Autodesk Fusion 360 part; units mm, degrees
(part 4 of 6)
sketch "minisub_split" plane through (0, 0, 0) normal (0, 1, 0) x (1, 0, 0)
  line L0 (140.6375, -31.1) -> (140.6375, -45.1)
  line L1 (169.2125, -12.05) -> (169.2125, -26.05)
  line L2 (135.5875, -31.1) -> (121.5875, -31.1)
  line L3 (64.4375, -45.1) -> (78.4375, -45.1)
  line L4 (97.4875, -31.1) -> (83.4875, -31.1)
  line L5 (164.1625, -26.05) -> (164.1625, -12.05)
  line L6 (140.6375, -45.1) -> (154.6375, -45.1)
  line L7 (78.4375, -31.1) -> (64.4375, -31.1)
  line L8 (150.1625, -12.05) -> (150.1625, -26.05)
  line L9 (59.3875, -45.1) -> (59.3875, -31.1)
  line L10 (135.5875, -45.1) -> (135.5875, -31.1)
  line L11 (212.075, -12.05) -> (212.075, -26.05)
  line L12 (0.1438, -45.1) -> (14.1438, -45.1)
  line L13 (14.1437, -31.1) -> (0.1437, -31.1)
  line L14 (121.5875, -31.1) -> (121.5875, -45.1)
  line L15 (83.4875, -31.1) -> (83.4875, -45.1)
  line L16 (64.4375, -31.1) -> (64.4375, -45.1)
  line L17 (45.3875, -31.1) -> (45.3875, -45.1)
  line L18 (154.6375, -45.1) -> (154.6375, -31.1)
  line L19 (183.2125, -12.05) -> (169.2125, -12.05)
  line L20 (14.1437, -45.1) -> (14.1437, -31.1)
  line L21 (126.0625, -26.05) -> (126.0625, -12.05)
  line L22 (93.0125, -12.05) -> (93.0125, -26.05)
  line L23 (0.1438, -31.1) -> (0.1438, -45.1)
  line L24 (112.0625, -26.05) -> (126.0625, -26.05)
  line L25 (212.075, -26.05) -> (226.075, -26.05)
  line L26 (126.0625, -12.05) -> (112.0625, -12.05)
  line L27 (173.6875, -31.1) -> (159.6875, -31.1)
  line L28 (159.6875, -45.1) -> (173.6875, -45.1)
  line L29 (73.9625, -12.05) -> (73.9625, -26.05)
  line L30 (40.3375, -45.1) -> (40.3375, -31.1)
  line L31 (169.2125, -26.05) -> (183.2125, -26.05)
  line L32 (26.3375, -45.1) -> (40.3375, -45.1)
  line L33 (131.1125, -26.05) -> (145.1125, -26.05)
  line L34 (107.0125, -12.05) -> (93.0125, -12.05)
  line L35 (45.3875, -45.1) -> (59.3875, -45.1)
  line L36 (188.2625, -12.05) -> (188.2625, -26.05)
  line L37 (116.5375, -45.1) -> (116.5375, -31.1)
  line L38 (115.5307, -49.15) -> (115.5307, -64.15)
  line L39 (171.3063, -50.15) -> (157.3063, -50.15)
  line L40 (78.4375, -45.1) -> (78.4375, -31.1)
  line L41 (202.2625, -12.05) -> (188.2625, -12.05)
  line L42 (226.075, -12.05) -> (212.075, -12.05)
  line L43 (145.1125, -12.05) -> (131.1125, -12.05)
  line L44 (226.075, -26.05) -> (226.075, -12.05)
  line L45 (216.8375, -64.15) -> (230.8375, -64.15)
  line L46 (159.6875, -31.1) -> (159.6875, -45.1)
  line L47 (90.3438, -50.15) -> (76.3438, -50.15)
  line L48 (76.3438, -50.15) -> (76.3438, -64.15)
  line L49 (137.9688, -50.15) -> (123.9688, -50.15)
  line L50 (98.7817, -64.15) -> (98.7817, -49.15)
  line L51 (98.7817, -49.15) -> (91.7817, -49.15)
  line L52 (230.8375, -45.1) -> (230.8375, -31.1)
  line L53 (123.9688, -50.15) -> (123.9688, -64.15)
  line L54 (197.7875, -45.1) -> (211.7875, -45.1)
  line L55 (230.8375, -50.15) -> (216.8375, -50.15)
  line L56 (197.7875, -31.1) -> (197.7875, -45.1)
  line L57 (122.5307, -49.15) -> (115.5307, -49.15)
  line L58 (30.8125, -50.15) -> (16.8125, -50.15)
  line L59 (9.3813, -50.15) -> (-4.6187, -50.15)
  line L60 (52.2438, -64.15) -> (52.2438, -50.15)
  line L61 (211.7875, -45.1) -> (211.7875, -31.1)
  line L62 (216.8375, -31.1) -> (216.8375, -45.1)
  line L63 (137.9688, -64.15) -> (137.9688, -50.15)
  line L64 (216.8375, -45.1) -> (230.8375, -45.1)
  line L65 (90.3438, -64.15) -> (90.3438, -50.15)
  line L66 (178.7375, -45.1) -> (192.7375, -45.1)
  line L67 (157.3063, -64.15) -> (171.3063, -64.15)
  line L68 (139.4067, -49.15) -> (139.4067, -64.15)
  line L69 (122.5307, -64.15) -> (122.5307, -49.15)
  line L70 (52.2438, -50.15) -> (38.2438, -50.15)
  line L71 (91.7817, -64.15) -> (98.7817, -64.15)
  line L72 (157.3063, -50.15) -> (157.3063, -64.15)
  line L73 (211.7875, -31.1) -> (197.7875, -31.1)
  line L74 (139.4067, -64.15) -> (146.4067, -64.15)
  line L75 (74.9058, -64.15) -> (74.9058, -49.15)
  line L76 (-4.6187, -64.15) -> (9.3813, -64.15)
  line L77 (178.7375, -31.1) -> (178.7375, -45.1)
  line L78 (67.9058, -49.15) -> (67.9058, -64.15)
  line L79 (178.7375, -64.15) -> (192.7375, -64.15)
  line L80 (197.7875, -64.15) -> (211.7875, -64.15)
  line L81 (211.7875, -50.15) -> (197.7875, -50.15)
  line L82 (211.7875, -64.15) -> (211.7875, -50.15)
  line L83 (74.9058, -49.15) -> (67.9058, -49.15)
  line L84 (38.2437, -64.15) -> (52.2438, -64.15)
  line L85 (192.7375, -31.1) -> (178.7375, -31.1)
  line L86 (192.7375, -45.1) -> (192.7375, -31.1)
  line L87 (16.8125, -64.15) -> (30.8125, -64.15)
  line L88 (171.3063, -64.15) -> (171.3063, -50.15)
  line L89 (192.7375, -50.15) -> (178.7375, -50.15)
  line L90 (230.8375, -31.1) -> (216.8375, -31.1)
  line L91 (16.8125, -50.15) -> (16.8125, -64.15)
  line L92 (67.9058, -64.15) -> (74.9058, -64.15)
  line L93 (192.7375, -64.15) -> (192.7375, -50.15)
  line L94 (123.9688, -64.15) -> (137.9688, -64.15)
  line L95 (9.3813, -64.15) -> (9.3813, -50.15)
  line L96 (178.7375, -50.15) -> (178.7375, -64.15)
  line L97 (173.6875, -45.1) -> (173.6875, -31.1)
  line L98 (91.7817, -49.15) -> (91.7817, -64.15)
  line L99 (146.4067, -49.15) -> (139.4067, -49.15)
  line L100 (146.4067, -64.15) -> (146.4067, -49.15)
  line L101 (115.5307, -64.15) -> (122.5307, -64.15)
  line L102 (76.3438, -64.15) -> (90.3438, -64.15)
  line L103 (230.8375, -64.15) -> (230.8375, -50.15)
  line L104 (-4.6187, -50.15) -> (-4.6187, -64.15)
  line L105 (216.8375, -50.15) -> (216.8375, -64.15)
  line L106 (197.7875, -50.15) -> (197.7875, -64.15)
  line L107 (38.2437, -50.15) -> (38.2437, -64.15)
  line L108 (30.8125, -64.15) -> (30.8125, -50.15)
  line L109 (-7, 7) -> (-7, -7)
  line L110 (31.1, 7) -> (31.1, -7)
  line L111 (121.3, 7) -> (107.3, 7)
  line L112 (107.3, 7) -> (107.3, -7)
  line L113 (69.2, -7) -> (83.2, -7)
  line L114 (102.25, 7) -> (88.25, 7)
  line L115 (107.3, -7) -> (121.3, -7)
  line L116 (145.4, 7) -> (145.4, -7)
  line L117 (12.05, 7) -> (12.05, -7)
  line L118 (50.15, -7) -> (64.15, -7)
  line L119 (64.15, 7) -> (50.15, 7)
  line L120 (26.05, -7) -> (26.05, 7)
  line L121 (26.05, 7) -> (12.05, 7)
  line L122 (64.15, -7) -> (64.15, 7)
  line L123 (45.1, 7) -> (31.1, 7)
  line L124 (121.3, -7) -> (121.3, 7)
  line L125 (140.35, -7) -> (140.35, 7)
  line L126 (159.4, 7) -> (145.4, 7)
  line L127 (88.25, 7) -> (88.25, -7)
  line L128 (7, -7) -> (7, 7)
  line L129 (50.15, 7) -> (50.15, -7)
  line L130 (178.45, 7) -> (164.45, 7)
  line L131 (126.35, -7) -> (140.35, -7)
  line L132 (12.05, -7) -> (26.05, -7)
  line L133 (-7, -7) -> (7, -7)
  line L134 (45.1, -7) -> (45.1, 7)
  line L135 (140.35, 7) -> (126.35, 7)
  line L136 (69.2, 7) -> (69.2, -7)
  line L137 (164.45, 7) -> (164.45, -7)
  line L138 (159.4, -7) -> (159.4, 7)
  line L139 (83.2, -7) -> (83.2, 7)
  line L140 (178.45, -7) -> (178.45, 7)
  line L141 (145.4, -7) -> (159.4, -7)
  line L142 (183.5, -7) -> (197.5, -7)
  line L143 (126.35, 7) -> (126.35, -7)
  line L144 (164.45, -7) -> (178.45, -7)
  line L145 (7, 7) -> (-7, 7)
  line L146 (88.25, -7) -> (102.25, -7)
  line L147 (31.1, -7) -> (45.1, -7)
  line L148 (102.25, -7) -> (102.25, 7)
  line L149 (83.2, 7) -> (69.2, 7)
  line L150 (183.5, 7) -> (183.5, -7)
  line L151 (209.6937, -7) -> (223.6938, -7)
  line L152 (223.6938, 7) -> (209.6937, 7)
  line L153 (223.6938, -7) -> (223.6938, 7)
  line L154 (209.6937, 7) -> (209.6937, -7)
  line L155 (197.5, 7) -> (183.5, 7)
  line L156 (197.5, -7) -> (197.5, 7)
  line L157 (-4.6187, -12.05) -> (-4.6187, -26.05)
  line L158 (16.8125, -26.05) -> (30.8125, -26.05)
  line L159 (30.8125, -12.05) -> (16.8125, -12.05)
  line L160 (30.8125, -26.05) -> (30.8125, -12.05)
  line L161 (35.8625, -26.05) -> (49.8625, -26.05)
  line L162 (35.8625, -12.05) -> (35.8625, -26.05)
  line L163 (68.9125, -26.05) -> (68.9125, -12.05)
  line L164 (54.9125, -12.05) -> (54.9125, -26.05)
  line L165 (73.9625, -26.05) -> (87.9625, -26.05)
  line L166 (49.8625, -26.05) -> (49.8625, -12.05)
  line L167 (68.9125, -12.05) -> (54.9125, -12.05)
  line L168 (54.9125, -26.05) -> (68.9125, -26.05)
  line L169 (9.3813, -12.05) -> (-4.6187, -12.05)
  line L170 (16.8125, -12.05) -> (16.8125, -26.05)
  line L171 (49.8625, -12.05) -> (35.8625, -12.05)
  line L172 (87.9625, -12.05) -> (73.9625, -12.05)
  line L173 (-4.6187, -26.05) -> (9.3813, -26.05)
  line L174 (9.3813, -26.05) -> (9.3813, -12.05)
  line L175 (107.0125, -26.05) -> (107.0125, -12.05)
  line L176 (202.2625, -26.05) -> (202.2625, -12.05)
  line L177 (26.3375, -31.1) -> (26.3375, -45.1)
  line L178 (150.1625, -26.05) -> (164.1625, -26.05)
  line L179 (83.4875, -45.1) -> (97.4875, -45.1)
  line L180 (121.5875, -45.1) -> (135.5875, -45.1)
  line L181 (183.2125, -26.05) -> (183.2125, -12.05)
  line L182 (154.6375, -31.1) -> (140.6375, -31.1)
  line L183 (131.1125, -12.05) -> (131.1125, -26.05)
  line L184 (112.0625, -12.05) -> (112.0625, -26.05)
  line L185 (40.3375, -31.1) -> (26.3375, -31.1)
  line L186 (102.5375, -45.1) -> (116.5375, -45.1)
  line L187 (97.4875, -45.1) -> (97.4875, -31.1)
  line L188 (87.9625, -26.05) -> (87.9625, -12.05)
  line L189 (93.0125, -26.05) -> (107.0125, -26.05)
  line L190 (102.5375, -31.1) -> (102.5375, -45.1)
  line L191 (116.5375, -31.1) -> (102.5375, -31.1)
  line L192 (145.1125, -26.05) -> (145.1125, -12.05)
  line L193 (188.2625, -26.05) -> (202.2625, -26.05)
  line L194 (59.3875, -31.1) -> (45.3875, -31.1)
  line L195 (164.1625, -12.05) -> (150.1625, -12.05)
sketch "m3n3van_r2" plane through (0, 0, 0) normal (0, 1, 0) x (1, 0, 0)
  line L0 (159.4, 7) -> (145.4, 7)
  line L1 (159.4, -7) -> (159.4, 7)
  line L2 (7, -7) -> (7, 7)
  line L3 (164.45, -7) -> (178.45, -7)
  line L4 (178.45, -7) -> (178.45, 7)
  line L5 (26.05, 7) -> (12.05, 7)
  line L6 (183.5, -7) -> (197.5, -7)
  line L7 (164.45, 7) -> (164.45, -7)
  line L8 (50.15, 7) -> (50.15, -7)
  line L9 (88.25, -7) -> (102.25, -7)
  line L10 (83.2, -7) -> (83.2, 7)
  line L11 (69.2, -7) -> (83.2, -7)
  line L12 (107.3, -7) -> (121.3, -7)
  line L13 (121.3, 7) -> (107.3, 7)
  line L14 (121.3, -7) -> (121.3, 7)
  line L15 (145.4, -7) -> (159.4, -7)
  line L16 (31.1, -7) -> (45.1, -7)
  line L17 (-7, 7) -> (-7, -7)
  line L18 (45.1, 7) -> (31.1, 7)
  line L19 (45.1, -7) -> (45.1, 7)
  line L20 (7, 7) -> (-7, 7)
  line L21 (12.05, 7) -> (12.05, -7)
  line L22 (178.45, 7) -> (164.45, 7)
  line L23 (145.4, 7) -> (145.4, -7)
  line L24 (26.05, -7) -> (26.05, 7)
  line L25 (102.25, 7) -> (88.25, 7)
  line L26 (50.15, -7) -> (64.15, -7)
  line L27 (126.35, 7) -> (126.35, -7)
  line L28 (-7, -7) -> (7, -7)
  line L29 (31.1, 7) -> (31.1, -7)
  line L30 (12.05, -7) -> (26.05, -7)
  line L31 (140.35, 7) -> (126.35, 7)
  line L32 (93.0125, -12.05) -> (93.0125, -26.05)
  line L33 (169.2125, -26.05) -> (183.2125, -26.05)
  line L34 (9.3812, -26.05) -> (9.3812, -12.05)
  line L35 (219.2187, -7) -> (223.6937, -7)
  line L36 (30.8125, -12.05) -> (16.8125, -12.05)
  line L37 (126.0625, -26.05) -> (126.0625, -12.05)
  line L38 (112.0625, -26.05) -> (126.0625, -26.05)
  line L39 (145.1125, -26.05) -> (145.1125, -12.05)
  line L40 (126.0625, -12.05) -> (112.0625, -12.05)
  line L41 (140.35, -7) -> (140.35, 7)
  line L42 (102.25, -7) -> (102.25, 7)
  line L43 (183.5, 7) -> (183.5, -7)
  line L44 (145.1125, -12.05) -> (131.1125, -12.05)
  line L45 (212.075, -26.05) -> (226.075, -26.05)
  line L46 (232.5253, 7) -> (223.6937, 7)
  line L47 (68.9125, -26.05) -> (68.9125, -12.05)
  line L48 (107.0125, -26.05) -> (107.0125, -12.05)
  line L49 (197.5, -7) -> (197.5, 7)
  line L50 (209.6937, -7) -> (216.55, -7)
  line L51 (49.8625, -12.05) -> (35.8625, -12.05)
  line L52 (83.2, 7) -> (69.2, 7)
  line L53 (107.0125, -12.05) -> (93.0125, -12.05)
  line L54 (164.1625, -12.05) -> (150.1625, -12.05)
  line L55 (150.1625, -12.05) -> (150.1625, -26.05)
  line L56 (223.6937, -7) -> (232.5253, -7)
  line L57 (188.2625, -26.05) -> (202.2625, -26.05)
  line L58 (16.8125, -12.05) -> (16.8125, -26.05)
  line L59 (223.6937, 7) -> (219.2187, 7)
  line L60 (209.6937, 7) -> (202.55, 7)
  line L61 (68.9125, -12.05) -> (54.9125, -12.05)
  line L62 (126.35, -7) -> (140.35, -7)
  line L63 (219.2187, 7) -> (216.55, 7)
  line L64 (216.55, 7) -> (209.6937, 7)
  line L65 (35.8625, -26.05) -> (49.8625, -26.05)
  line L66 (30.8125, -26.05) -> (30.8125, -12.05)
  line L67 (73.9625, -26.05) -> (87.9625, -26.05)
  line L68 (-4.6187, -12.05) -> (-4.6187, -26.05)
  line L69 (54.9125, -26.05) -> (68.9125, -26.05)
  line L70 (202.55, 7) -> (202.55, -7)
  line L71 (169.2125, -12.05) -> (169.2125, -26.05)
  line L72 (202.2625, -26.05) -> (202.2625, -12.05)
  line L73 (49.8625, -26.05) -> (49.8625, -12.05)
  line L74 (112.0625, -12.05) -> (112.0625, -26.05)
  line L75 (131.1125, -26.05) -> (145.1125, -26.05)
  line L76 (131.1125, -12.05) -> (131.1125, -26.05)
  line L77 (107.3, 7) -> (107.3, -7)
  line L78 (216.55, -7) -> (219.2187, -7)
  line L79 (-4.6187, -26.05) -> (9.3812, -26.05)
  line L80 (16.8125, -26.05) -> (30.8125, -26.05)
  line L81 (54.9125, -12.05) -> (54.9125, -26.05)
  line L82 (64.15, -7) -> (64.15, 7)
  line L83 (197.5, 7) -> (183.5, 7)
  line L84 (64.15, 7) -> (50.15, 7)
  line L85 (87.9625, -26.05) -> (87.9625, -12.05)
  line L86 (35.8625, -12.05) -> (35.8625, -26.05)
  line L87 (202.2625, -12.05) -> (188.2625, -12.05)
  line L88 (183.2125, -12.05) -> (169.2125, -12.05)
  line L89 (183.2125, -26.05) -> (183.2125, -12.05)
  line L90 (9.3812, -12.05) -> (-4.6187, -12.05)
  line L91 (188.2625, -12.05) -> (188.2625, -26.05)
  line L92 (88.25, 7) -> (88.25, -7)
  line L93 (202.55, -7) -> (209.6937, -7)
  line L94 (69.2, 7) -> (69.2, -7)
  line L95 (232.5253, -7) -> (232.5253, 7)
  line L96 (87.9625, -12.05) -> (73.9625, -12.05)
  line L97 (64.4375, -31.1) -> (64.4375, -45.1)
  line L98 (216.8375, -31.1) -> (216.8375, -45.1)
  line L99 (14.1437, -45.1) -> (14.1437, -31.1)
  line L100 (14.4313, -64.15) -> (28.4312, -64.15)
  line L101 (40.3375, -31.1) -> (26.3375, -31.1)
  line L102 (59.3875, -31.1) -> (45.3875, -31.1)
  line L103 (102.5375, -45.1) -> (116.5375, -45.1)
  line L104 (230.8375, -45.1) -> (230.8375, -31.1)
  line L105 (164.1625, -26.05) -> (164.1625, -12.05)
  line L106 (121.5875, -31.1) -> (121.5875, -45.1)
  line L107 (7, -50.15) -> (-7, -50.15)
  line L108 (116.5375, -31.1) -> (102.5375, -31.1)
  line L109 (211.7875, -45.1) -> (211.7875, -31.1)
  line L110 (28.4312, -50.15) -> (14.4313, -50.15)
  line L111 (140.6375, -45.1) -> (154.6375, -45.1)
  line L112 (102.5375, -31.1) -> (102.5375, -45.1)
  line L113 (135.5875, -31.1) -> (121.5875, -31.1)
  line L114 (14.4313, -50.15) -> (14.4313, -64.15)
  line L115 (26.3375, -31.1) -> (26.3375, -45.1)
  line L116 (78.4375, -31.1) -> (64.4375, -31.1)
  line L117 (192.7375, -31.1) -> (178.7375, -31.1)
  line L118 (73.9625, -12.05) -> (73.9625, -26.05)
  line L119 (197.7875, -45.1) -> (211.7875, -45.1)
  line L120 (78.4375, -45.1) -> (78.4375, -31.1)
  line L121 (28.4312, -64.15) -> (28.4312, -50.15)
  line L122 (0.1438, -31.1) -> (0.1438, -45.1)
  line L123 (73.9625, -64.15) -> (87.9625, -64.15)
  line L124 (159.6875, -31.1) -> (159.6875, -45.1)
  line L125 (150.1625, -26.05) -> (164.1625, -26.05)
  line L126 (173.6875, -45.1) -> (173.6875, -31.1)
  line L127 (226.075, -26.05) -> (226.075, -12.05)
  line L128 (197.7875, -31.1) -> (197.7875, -45.1)
  line L129 (14.1437, -31.1) -> (0.1438, -31.1)
  line L130 (35.8625, -50.15) -> (35.8625, -64.15)
  line L131 (49.8625, -64.15) -> (49.8625, -50.15)
  line L132 (97.4875, -31.1) -> (83.4875, -31.1)
  line L133 (97.4875, -45.1) -> (97.4875, -31.1)
  line L134 (121.5875, -45.1) -> (135.5875, -45.1)
  line L135 (35.8625, -64.15) -> (49.8625, -64.15)
  line L136 (226.075, -12.05) -> (212.075, -12.05)
  line L137 (173.6875, -31.1) -> (159.6875, -31.1)
  line L138 (211.7875, -31.1) -> (197.7875, -31.1)
  line L139 (192.7375, -45.1) -> (192.7375, -31.1)
  line L140 (49.8625, -50.15) -> (35.8625, -50.15)
  line L141 (64.4375, -45.1) -> (78.4375, -45.1)
  line L142 (-7, -50.15) -> (-7, -64.15)
  line L143 (93.0125, -26.05) -> (107.0125, -26.05)
  line L144 (83.4875, -31.1) -> (83.4875, -45.1)
  line L145 (154.6375, -45.1) -> (154.6375, -31.1)
  line L146 (26.3375, -45.1) -> (40.3375, -45.1)
  line L147 (45.3875, -45.1) -> (59.3875, -45.1)
  line L148 (45.3875, -31.1) -> (45.3875, -45.1)
  line L149 (116.5375, -45.1) -> (116.5375, -31.1)
  line L150 (83.4875, -45.1) -> (97.4875, -45.1)
  line L151 (154.6375, -31.1) -> (140.6375, -31.1)
  line L152 (230.8375, -31.1) -> (216.8375, -31.1)
  line L153 (178.7375, -45.1) -> (192.7375, -45.1)
  line L154 (7, -64.15) -> (7, -50.15)
  line L155 (178.7375, -31.1) -> (178.7375, -45.1)
  line L156 (0.1438, -45.1) -> (14.1437, -45.1)
  line L157 (216.8375, -45.1) -> (230.8375, -45.1)
  line L158 (212.075, -12.05) -> (212.075, -26.05)
  line L159 (140.6375, -31.1) -> (140.6375, -45.1)
  line L160 (-7, -64.15) -> (7, -64.15)
  line L161 (115.5625, -64.15) -> (122.5625, -64.15)
  line L162 (87.9625, -64.15) -> (87.9625, -50.15)
  line L163 (185.5937, -50.15) -> (171.5937, -50.15)
  line L164 (214.4562, -50.15) -> (214.4562, -64.15)
  line L165 (131.1125, -50.15) -> (131.1125, -64.15)
  line L166 (171.5937, -50.15) -> (171.5937, -64.15)
  line L167 (207.025, -50.15) -> (193.025, -50.15)
  line L168 (65.4125, -49.15) -> (58.4125, -49.15)
  line L169 (115.5625, -49.15) -> (115.5625, -64.15)
  line L170 (228.4562, -64.15) -> (228.4562, -50.15)
  line L171 (160.6625, -64.15) -> (160.6625, -49.15)
  line L172 (103.5125, -64.15) -> (103.5125, -49.15)
  line L173 (145.1125, -64.15) -> (145.1125, -50.15)
  line L174 (193.025, -64.15) -> (207.025, -64.15)
  line L175 (59.3875, -45.1) -> (59.3875, -31.1)
  line L176 (122.5625, -49.15) -> (115.5625, -49.15)
  line L177 (145.1125, -50.15) -> (131.1125, -50.15)
  line L178 (103.5125, -49.15) -> (96.5125, -49.15)
  line L179 (131.1125, -64.15) -> (145.1125, -64.15)
  line L180 (159.6875, -45.1) -> (173.6875, -45.1)
  line L181 (40.3375, -45.1) -> (40.3375, -31.1)
  line L182 (135.5875, -45.1) -> (135.5875, -31.1)
  line L183 (160.6625, -49.15) -> (153.6625, -49.15)
  line L184 (96.5125, -64.15) -> (103.5125, -64.15)
  line L185 (171.5937, -64.15) -> (185.5937, -64.15)
  line L186 (193.025, -50.15) -> (193.025, -64.15)
  line L187 (214.4562, -64.15) -> (228.4562, -64.15)
  line L188 (65.4125, -64.15) -> (65.4125, -49.15)
  line L189 (122.5625, -64.15) -> (122.5625, -49.15)
  line L190 (185.5937, -64.15) -> (185.5937, -50.15)
  line L191 (73.9625, -50.15) -> (73.9625, -64.15)
  line L192 (96.5125, -49.15) -> (96.5125, -64.15)
  line L193 (87.9625, -50.15) -> (73.9625, -50.15)
  line L194 (153.6625, -49.15) -> (153.6625, -64.15)
  line L195 (228.4562, -50.15) -> (214.4562, -50.15)
  line L196 (153.6625, -64.15) -> (160.6625, -64.15)
  line L197 (58.4125, -64.15) -> (65.4125, -64.15)
  line L198 (207.025, -64.15) -> (207.025, -50.15)
  line L199 (58.4125, -49.15) -> (58.4125, -64.15)
sketch "asymptote" plane through (0, 0, 0) normal (0, 1, 0) x (1, 0, 0)
  line L0 (54.9125, -26.05) -> (54.9125, -12.05)
  line L1 (97.4875, -31.1) -> (97.4875, -45.1)
  line L2 (97.4875, -45.1) -> (83.4875, -45.1)
  line L3 (83.4875, -45.1) -> (83.4875, -31.1)
  line L4 (71.2938, -64.15) -> (57.2938, -64.15)
  line L5 (107.3, 7) -> (121.3, 7)
  line L6 (121.3, 7) -> (121.3, -7)
  line L7 (121.3, -7) -> (107.3, -7)
  line L8 (107.3, -7) -> (107.3, 7)
  line L9 (145.1125, -12.05) -> (145.1125, -26.05)
  line L10 (57.2938, -64.15) -> (57.2938, -50.15)
  line L11 (145.1125, -26.05) -> (131.1125, -26.05)
  line L12 (131.1125, -26.05) -> (131.1125, -12.05)
  line L13 (58.4125, -49.15) -> (65.4125, -49.15)
  line L14 (7, 7) -> (7, -7)
  line L15 (40.3375, -31.1) -> (40.3375, -45.1)
  line L16 (26.3375, -31.1) -> (40.3375, -31.1)
  line L17 (54.9125, -12.05) -> (68.9125, -12.05)
  line L18 (68.9125, -12.05) -> (68.9125, -26.05)
  line L19 (40.3375, -45.1) -> (26.3375, -45.1)
  line L20 (71.2938, -50.15) -> (71.2938, -64.15)
  line L21 (57.2938, -50.15) -> (58.4125, -50.15)
  line L22 (65.4125, -50.15) -> (71.2938, -50.15)
  line L23 (65.4125, -49.15) -> (65.4125, -50.15)
  line L24 (26.3375, -45.1) -> (26.3375, -31.1)
  line L25 (7, -7) -> (-7, -7)
  line L26 (-7, -7) -> (-7, 7)
  line L27 (68.9125, -26.05) -> (54.9125, -26.05)
  line L28 (58.4125, -50.15) -> (58.4125, -49.15)
  line L29 (-7, 7) -> (7, 7)
  line L30 (83.4875, -31.1) -> (97.4875, -31.1)
  line L31 (50.15, 7) -> (64.15, 7)
  line L32 (230.8375, -31.1) -> (230.8375, -45.1)
  line L33 (-4.6187, -12.05) -> (9.3812, -12.05)
  line L34 (49.8625, -12.05) -> (49.8625, -26.05)
  line L35 (226.075, -12.05) -> (226.075, -26.05)
  line L36 (188.2625, -12.05) -> (202.2625, -12.05)
  line L37 (9.3812, -26.05) -> (-4.6187, -26.05)
  line L38 (50.15, -7) -> (50.15, 7)
  line L39 (192.7375, -45.1) -> (178.7375, -45.1)
  line L40 (88.25, -7) -> (88.25, 7)
  line L41 (159.6875, -45.1) -> (159.6875, -31.1)
  line L42 (9.3812, -12.05) -> (9.3812, -26.05)
  line L43 (-4.6187, -26.05) -> (-4.6187, -12.05)
  line L44 (37.9563, -64.15) -> (-2.2375, -64.15)
  line L45 (226.075, -26.05) -> (212.075, -26.05)
  line L46 (230.8375, -45.1) -> (216.8375, -45.1)
  line L47 (183.2125, -12.05) -> (183.2125, -26.05)
  line L48 (103.5125, -49.15) -> (103.5125, -50.15)
  line L49 (88.25, 7) -> (102.25, 7)
  line L50 (216.8375, -31.1) -> (230.8375, -31.1)
  line L51 (192.7375, -31.1) -> (192.7375, -45.1)
  line L52 (173.6875, -45.1) -> (159.6875, -45.1)
  line L53 (131.1125, -12.05) -> (145.1125, -12.05)
  line L54 (159.6875, -31.1) -> (173.6875, -31.1)
  line L55 (173.6875, -31.1) -> (173.6875, -45.1)
  line L56 (178.7375, -31.1) -> (192.7375, -31.1)
  line L57 (212.075, -26.05) -> (212.075, -12.05)
  line L58 (188.2625, -26.05) -> (188.2625, -12.05)
  line L59 (64.15, 7) -> (64.15, -7)
  line L60 (32.1068, -50.15) -> (37.9563, -50.15)
  line L61 (73.9625, -64.15) -> (73.9625, -50.15)
  line L62 (169.2125, -26.05) -> (169.2125, -12.05)
  line L63 (12.05, 7) -> (26.05, 7)
  line L64 (26.05, 7) -> (26.05, -7)
  line L65 (25.1068, -50.15) -> (25.1068, -49.15)
  line L66 (64.4375, -31.1) -> (78.4375, -31.1)
  line L67 (32.1068, -49.15) -> (32.1068, -50.15)
  line L68 (-2.2375, -64.15) -> (-2.2375, -50.15)
  line L69 (122.5625, -49.15) -> (122.5625, -50.15)
  line L70 (145.1125, -50.15) -> (145.1125, -64.15)
  line L71 (216.8375, -45.1) -> (216.8375, -31.1)
  line L72 (178.7375, -45.1) -> (178.7375, -31.1)
  line L73 (212.075, -12.05) -> (226.075, -12.05)
  line L74 (-2.2375, -50.15) -> (1.2308, -50.15)
  line L75 (202.2625, -12.05) -> (202.2625, -26.05)
  line L76 (202.2625, -26.05) -> (188.2625, -26.05)
  line L77 (140.6375, -45.1) -> (140.6375, -31.1)
  line L78 (64.15, -7) -> (50.15, -7)
  line L79 (8.2307, -50.15) -> (25.1068, -50.15)
  line L80 (112.0625, -26.05) -> (112.0625, -12.05)
  line L81 (35.8625, -12.05) -> (49.8625, -12.05)
  line L82 (1.2308, -49.15) -> (8.2307, -49.15)
  line L83 (122.5625, -50.15) -> (145.1125, -50.15)
  line L84 (169.2125, -12.05) -> (183.2125, -12.05)
  line L85 (73.9625, -50.15) -> (96.5125, -50.15)
  line L86 (35.8625, -26.05) -> (35.8625, -12.05)
  line L87 (83.2, 7) -> (83.2, -7)
  line L88 (96.5125, -50.15) -> (96.5125, -49.15)
  line L89 (1.2308, -50.15) -> (1.2308, -49.15)
  line L90 (78.4375, -45.1) -> (64.4375, -45.1)
  line L91 (96.5125, -49.15) -> (103.5125, -49.15)
  line L92 (140.6375, -31.1) -> (154.6375, -31.1)
  line L93 (126.0625, -26.05) -> (112.0625, -26.05)
  line L94 (83.2, -7) -> (69.2, -7)
  line L95 (145.4, -7) -> (145.4, 7)
  line L96 (197.5, 7) -> (197.5, -7)
  line L97 (197.7875, -45.1) -> (197.7875, -31.1)
  line L98 (37.9563, -50.15) -> (37.9563, -64.15)
  line L99 (145.1125, -64.15) -> (73.9625, -64.15)
  line L100 (78.4375, -31.1) -> (78.4375, -45.1)
  line L101 (14.1437, -31.1) -> (14.1437, -45.1)
  line L102 (49.8625, -26.05) -> (35.8625, -26.05)
  line L103 (112.0625, -12.05) -> (126.0625, -12.05)
  line L104 (107.0125, -26.05) -> (93.0125, -26.05)
  line L105 (189.2375, -49.15) -> (189.2375, -50.15)
  line L106 (8.2307, -49.15) -> (8.2307, -50.15)
  line L107 (183.2125, -26.05) -> (169.2125, -26.05)
  line L108 (64.4375, -45.1) -> (64.4375, -31.1)
  line L109 (0.1438, -45.1) -> (0.1438, -31.1)
  line L110 (93.0125, -26.05) -> (93.0125, -12.05)
  line L111 (154.6375, -45.1) -> (140.6375, -45.1)
  line L112 (154.6375, -31.1) -> (154.6375, -45.1)
  line L113 (126.0625, -12.05) -> (126.0625, -26.05)
  line L114 (12.05, -7) -> (12.05, 7)
  line L115 (227.3375, -50.15) -> (230.8375, -50.15)
  line L116 (126.35, -7) -> (126.35, 7)
  line L117 (26.05, -7) -> (12.05, -7)
  line L118 (209.6938, -7) -> (209.6938, 7)
  line L119 (140.35, -7) -> (126.35, -7)
  line L120 (69.2, 7) -> (83.2, 7)
  line L121 (0.1438, -31.1) -> (14.1437, -31.1)
  line L122 (14.1437, -45.1) -> (0.1438, -45.1)
  line L123 (115.5625, -50.15) -> (115.5625, -49.15)
  line L124 (103.5125, -50.15) -> (115.5625, -50.15)
  line L125 (25.1068, -49.15) -> (32.1068, -49.15)
  line L126 (102.25, -7) -> (88.25, -7)
  line L127 (115.5625, -49.15) -> (122.5625, -49.15)
  line L128 (102.5375, -45.1) -> (102.5375, -31.1)
  line L129 (102.25, 7) -> (102.25, -7)
  line L130 (164.1625, -26.05) -> (150.1625, -26.05)
  line L131 (211.7875, -31.1) -> (211.7875, -45.1)
  line L132 (116.5375, -45.1) -> (102.5375, -45.1)
  line L133 (211.7875, -45.1) -> (197.7875, -45.1)
  line L134 (223.6938, 7) -> (223.6938, -7)
  line L135 (178.7375, -50.15) -> (182.2375, -50.15)
  line L136 (159.4, 7) -> (159.4, -7)
  line L137 (150.1625, -26.05) -> (150.1625, -12.05)
  line L138 (182.2375, -50.15) -> (182.2375, -49.15)
  line L139 (31.1, -7) -> (31.1, 7)
  line L140 (189.2375, -50.15) -> (220.3375, -50.15)
  line L141 (220.3375, -50.15) -> (220.3375, -49.15)
  line L142 (230.8375, -50.15) -> (230.8375, -64.15)
  line L143 (178.45, 7) -> (178.45, -7)
  line L144 (135.5875, -31.1) -> (135.5875, -45.1)
  line L145 (87.9625, -26.05) -> (73.9625, -26.05)
  line L146 (182.2375, -49.15) -> (189.2375, -49.15)
  line L147 (45.1, 7) -> (45.1, -7)
  line L148 (102.5375, -31.1) -> (116.5375, -31.1)
  line L149 (178.7375, -64.15) -> (178.7375, -50.15)
  line L150 (150.1625, -12.05) -> (164.1625, -12.05)
  line L151 (69.2, -7) -> (69.2, 7)
  line L152 (73.9625, -12.05) -> (87.9625, -12.05)
  line L153 (178.45, -7) -> (164.45, -7)
  line L154 (197.7875, -31.1) -> (211.7875, -31.1)
  line L155 (230.8375, -64.15) -> (178.7375, -64.15)
  line L156 (164.45, -7) -> (164.45, 7)
  line L157 (209.6938, 7) -> (223.6938, 7)
  line L158 (183.5, -7) -> (183.5, 7)
  line L159 (220.3375, -49.15) -> (227.3375, -49.15)
  line L160 (45.1, -7) -> (31.1, -7)
  line L161 (31.1, 7) -> (45.1, 7)
  line L162 (87.9625, -12.05) -> (87.9625, -26.05)
  line L163 (183.5, 7) -> (197.5, 7)
  line L164 (223.6938, -7) -> (209.6938, -7)
  line L165 (121.5875, -31.1) -> (135.5875, -31.1)
  line L166 (93.0125, -12.05) -> (107.0125, -12.05)
  line L167 (227.3375, -49.15) -> (227.3375, -50.15)
  line L168 (145.4, 7) -> (159.4, 7)
  line L169 (140.35, 7) -> (140.35, -7)
  line L170 (135.5875, -45.1) -> (121.5875, -45.1)
  line L171 (107.0125, -12.05) -> (107.0125, -26.05)
  line L172 (197.5, -7) -> (183.5, -7)
  line L173 (73.9625, -26.05) -> (73.9625, -12.05)
  line L174 (126.35, 7) -> (140.35, 7)
  line L175 (164.45, 7) -> (178.45, 7)
  line L176 (116.5375, -31.1) -> (116.5375, -45.1)
  line L177 (159.4, -7) -> (145.4, -7)
  line L178 (164.1625, -12.05) -> (164.1625, -26.05)
  line L179 (121.5875, -45.1) -> (121.5875, -31.1)
  line L180 (30.8125, -12.05) -> (30.8125, -26.05)
  line L181 (153.6625, -49.15) -> (160.6625, -49.15)
  line L182 (16.8125, -12.05) -> (30.8125, -12.05)
  line L183 (45.3875, -45.1) -> (45.3875, -31.1)
  line L184 (147.7813, -50.15) -> (153.6625, -50.15)
  line L185 (45.3875, -31.1) -> (59.3875, -31.1)
  line L186 (160.6625, -50.15) -> (161.7813, -50.15)
  line L187 (30.8125, -26.05) -> (16.8125, -26.05)
  line L188 (153.6625, -50.15) -> (153.6625, -49.15)
  line L189 (59.3875, -31.1) -> (59.3875, -45.1)
  line L190 (161.7813, -50.15) -> (161.7813, -64.15)
  line L191 (160.6625, -49.15) -> (160.6625, -50.15)
  line L192 (16.8125, -26.05) -> (16.8125, -12.05)
  line L193 (59.3875, -45.1) -> (45.3875, -45.1)
  line L194 (161.7813, -64.15) -> (147.7813, -64.15)
  line L195 (147.7813, -64.15) -> (147.7813, -50.15)
sketch "asymptote_7u" plane through (35.5023, 0, -36.9816) normal (0, 1, 0) x (1, 0, 0)
  line L0 (81.0349, -96.4308) -> (127.8099, -96.4308)
  line L1 (134.5609, -96.4308) -> (135.3849, -96.4308)
  line L2 (13.5097, -87.3619) -> (13.5097, -93.632)
  line L3 (67.0356, -96.4322) -> (67.0356, -101.1313)
  line L4 (15.235, -86.1616) -> (15.235, -87.3619)
  line L5 (18.5341, -87.3619) -> (18.5341, -86.1616)
  line L6 (135.3849, -96.4308) -> (135.3849, -93.6306)
  line L7 (129.5349, -86.1603) -> (129.5349, -87.3605)
  line L8 (129.5349, -87.3605) -> (127.8099, -87.3605)
  line L9 (132.8349, -87.3605) -> (132.8349, -86.1603)
  line L10 (134.5609, -93.6306) -> (134.5609, -87.3605)
  line L11 (18.5341, -86.1616) -> (15.235, -86.1616)
  line L12 (12.6843, -96.4322) -> (13.5097, -96.4322)
  line L13 (127.8099, -99.6623) -> (134.5609, -99.6623)
  line L14 (134.5609, -87.3605) -> (132.8349, -87.3605)
  line L15 (135.3849, -93.6306) -> (134.5609, -93.6306)
  line L16 (20.2608, -99.6623) -> (20.2608, -96.4322)
  line L17 (127.8099, -87.3605) -> (127.8099, -91.8309)
  line L18 (134.5609, -99.6623) -> (134.5609, -96.4308)
  line L19 (81.0349, -87.1318) -> (67.0356, -87.1318)
  line L20 (12.6843, -93.632) -> (12.6843, -96.4322)
  line L21 (67.0356, -87.1318) -> (67.0356, -91.8323)
  line L22 (13.5097, -93.632) -> (12.6843, -93.632)
  line L23 (20.2608, -87.3619) -> (18.5341, -87.3619)
  line L24 (127.8099, -91.8309) -> (81.0349, -91.8309)
  line L25 (15.235, -87.3619) -> (13.5097, -87.3619)
  line L26 (67.0356, -101.1313) -> (81.0349, -101.1313)
  line L27 (20.2608, -91.8323) -> (20.2608, -87.3619)
  line L28 (132.8349, -86.1603) -> (129.5349, -86.1603)
  line L29 (67.0356, -91.8323) -> (20.2608, -91.8323)
  line L30 (13.5097, -96.4322) -> (13.5097, -99.6623)
  line L31 (81.0349, -101.1313) -> (81.0349, -96.4308)
  line L32 (81.0349, -91.8309) -> (81.0349, -87.1318)
  line L33 (20.2608, -96.4322) -> (67.0356, -96.4322)
  line L34 (127.8099, -96.4308) -> (127.8099, -99.6623)
  line L35 (13.5097, -99.6623) -> (20.2608, -99.6623)
  line L36 (67.0356, -87.1318) -> (81.0349, -101.1313) construction
  line L37 (67.0356, -101.1313) -> (81.0349, -87.1318) construction
sketch "minibaen" plane through (0, 0, 0) normal (0, 1, 0) x (1, 0, 0)
  line L0 (104.919, -31.098) -> (104.919, -45.098)
  line L1 (118.919, -45.098) -> (118.919, -31.098)
  line L2 (67.559, -64.148) -> (68.461, -64.148)
  line L3 (160.959, -31.098) -> (160.959, -45.098)
  line L4 (216.999, -31.098) -> (216.999, -45.098)
  line L5 (86.239, -31.098) -> (86.239, -45.098)
  line L6 (160.959, -45.098) -> (174.959, -45.098)
  line L7 (81.559, -50.148) -> (76.899, -50.148)
  line L8 (90.109, -64.148) -> (90.899, -64.148)
  line L9 (25.519, -64.148) -> (25.519, -50.148)
  line L10 (198.319, -31.098) -> (198.319, -45.098)
  line L11 (230.999, -45.098) -> (230.999, -31.098)
  line L12 (137.599, -50.148) -> (133.729, -50.148)
  line L13 (124.501, -64.148) -> (126.729, -64.148)
  line L14 (172.569, -49.148) -> (171.829, -49.148)
  line L15 (48.879, -64.148) -> (51.269, -64.148)
  line L16 (179.639, -31.098) -> (179.639, -45.098)
  line L17 (148.377, -49.148) -> (148.377, -50.148)
  line L18 (59.009, -64.148) -> (62.879, -64.148)
  line L19 (76.899, -64.148) -> (81.559, -64.148)
  line L20 (52.009, -64.148) -> (58.269, -64.148)
  line L21 (68.461, -50.148) -> (67.559, -50.148)
  line L22 (165.569, -49.148) -> (164.829, -49.148)
  line L23 (118.919, -64.148) -> (118.919, -50.148)
  line L24 (164.829, -64.148) -> (165.569, -64.148)
  line L25 (90.109, -50.148) -> (86.239, -50.148)
  line L26 (86.239, -64.148) -> (90.109, -64.148)
  line L27 (146.939, -64.148) -> (148.377, -64.148)
  line L28 (104.919, -50.148) -> (104.919, -64.148)
  line L29 (97.109, -64.148) -> (99.337, -64.148)
  line L30 (126.729, -49.148) -> (124.501, -49.148)
  line L31 (123.599, -45.098) -> (137.599, -45.098)
  line L32 (193.639, -45.098) -> (193.639, -31.098)
  line L33 (-7.161, -64.148) -> (6.839, -64.148)
  line L34 (58.269, -64.148) -> (59.009, -64.148)
  line L35 (30.199, -50.148) -> (30.199, -64.148)
  line L36 (59.009, -50.148) -> (59.009, -49.148)
  line L37 (212.319, -45.098) -> (212.319, -31.098)
  line L38 (137.599, -45.098) -> (137.599, -31.098)
  line L39 (133.729, -64.148) -> (137.599, -64.148)
  line L40 (146.939, -50.148) -> (142.279, -50.148)
  line L41 (100.239, -31.098) -> (86.239, -31.098)
  line L42 (142.279, -50.148) -> (137.599, -50.148)
  line L43 (-7.161, -50.148) -> (-7.161, -64.148)
  line L44 (230.999, -31.098) -> (216.999, -31.098)
  line L45 (126.729, -64.148) -> (131.501, -64.148)
  line L46 (156.279, -50.148) -> (155.377, -50.148)
  line L47 (124.501, -49.148) -> (124.501, -50.148)
  line L48 (133.729, -49.148) -> (131.501, -49.148)
  line L49 (155.377, -64.148) -> (156.279, -64.148)
  line L50 (142.279, -64.148) -> (146.939, -64.148)
  line L51 (48.879, -50.148) -> (48.879, -64.148)
  line L52 (86.239, -50.148) -> (81.559, -50.148)
  line L53 (131.501, -64.148) -> (132.939, -64.148)
  line L54 (123.599, -50.148) -> (123.599, -64.148)
  line L55 (148.377, -50.148) -> (146.939, -50.148)
  line L56 (124.501, -50.148) -> (123.599, -50.148)
  line L57 (160.959, -64.148) -> (164.829, -64.148)
  line L58 (172.569, -64.148) -> (174.959, -64.148)
  line L59 (174.959, -50.148) -> (172.569, -50.148)
  line L60 (171.829, -64.148) -> (172.569, -64.148)
  line L61 (68.461, -49.148) -> (68.461, -50.148)
  line L62 (104.919, -64.148) -> (118.919, -64.148)
  line L63 (179.639, -50.148) -> (179.639, -64.148)
  line L64 (52.009, -49.148) -> (51.269, -49.148)
  line L65 (164.829, -49.148) -> (164.829, -50.148)
  line L66 (75.461, -50.148) -> (75.461, -49.148)
  line L67 (171.829, -49.148) -> (165.569, -49.148)
  line L68 (164.829, -50.148) -> (160.959, -50.148)
  line L69 (132.939, -64.148) -> (133.729, -64.148)
  line L70 (81.559, -64.148) -> (86.239, -64.148)
  line L71 (99.337, -49.148) -> (97.109, -49.148)
  line L72 (131.501, -49.148) -> (126.729, -49.148)
  line L73 (155.377, -50.148) -> (155.377, -49.148)
  line L74 (156.279, -64.148) -> (156.279, -50.148)
  line L75 (174.959, -64.148) -> (174.959, -50.148)
  line L76 (51.269, -49.148) -> (51.269, -50.148)
  line L77 (148.377, -64.148) -> (155.377, -64.148)
  line L78 (99.337, -50.148) -> (99.337, -49.148)
  line L79 (100.239, -50.148) -> (99.337, -50.148)
  line L80 (230.999, -64.148) -> (230.999, -50.148)
  line L81 (51.269, -50.148) -> (48.879, -50.148)
  line L82 (100.239, -64.148) -> (100.239, -50.148)
  line L83 (212.319, -50.148) -> (198.319, -50.148)
  line L84 (198.319, -50.148) -> (198.319, -64.148)
  line L85 (75.461, -49.148) -> (68.461, -49.148)
  line L86 (179.639, -64.148) -> (193.639, -64.148)
  line L87 (212.319, -64.148) -> (212.319, -50.148)
  line L88 (198.319, -64.148) -> (212.319, -64.148)
  line L89 (165.569, -64.148) -> (171.829, -64.148)
  line L90 (99.337, -64.148) -> (100.239, -64.148)
  line L91 (230.999, -50.148) -> (216.999, -50.148)
  line L92 (155.377, -49.148) -> (148.377, -49.148)
  line L93 (62.879, -64.148) -> (62.879, -50.148)
  line L94 (62.879, -50.148) -> (59.009, -50.148)
  line L95 (118.919, -50.148) -> (104.919, -50.148)
  line L96 (172.569, -50.148) -> (172.569, -49.148)
  line L97 (216.999, -64.148) -> (230.999, -64.148)
  line L98 (160.959, -50.148) -> (160.959, -64.148)
  line L99 (193.639, -64.148) -> (193.639, -50.148)
  line L100 (123.599, -64.148) -> (124.501, -64.148)
  line L101 (216.999, -50.148) -> (216.999, -64.148)
  line L102 (133.729, -50.148) -> (133.729, -49.148)
  line L103 (137.599, -64.148) -> (142.279, -64.148)
  line L104 (193.639, -50.148) -> (179.639, -50.148)
  line L105 (216.999, -12.048) -> (216.999, -26.048)
  line L106 (62.879, -26.048) -> (62.879, -12.048)
  line L107 (104.919, -45.098) -> (118.919, -45.098)
  line L108 (67.559, -50.148) -> (67.559, -64.148)
  line L109 (137.599, -31.098) -> (123.599, -31.098)
  line L110 (44.199, -64.148) -> (44.199, -50.148)
  line L111 (142.279, -12.048) -> (142.279, -26.048)
  line L112 (11.519, -64.148) -> (25.519, -64.148)
  line L113 (193.639, -31.098) -> (179.639, -31.098)
  line L114 (67.559, -12.048) -> (67.559, -26.048)
  line L115 (100.239, -12.048) -> (86.239, -12.048)
  line L116 (137.599, -12.048) -> (123.599, -12.048)
  line L117 (86.239, -12.048) -> (86.239, -26.048)
  line L118 (118.919, -12.048) -> (104.919, -12.048)
  line L119 (174.959, -12.048) -> (160.959, -12.048)
  line L120 (100.239, -26.048) -> (100.239, -12.048)
  line L121 (179.639, -12.048) -> (179.639, -26.048)
  line L122 (62.879, -45.098) -> (62.879, -31.098)
  line L123 (123.599, -12.048) -> (123.599, -26.048)
  line L124 (67.559, -26.048) -> (81.559, -26.048)
  line L125 (11.519, -50.148) -> (11.519, -64.148)
  line L126 (142.279, -26.048) -> (156.279, -26.048)
  line L127 (156.279, -26.048) -> (156.279, -12.048)
  line L128 (30.199, -31.098) -> (30.199, -45.098)
  line L129 (86.239, -45.098) -> (100.239, -45.098)
  line L130 (212.319, -26.048) -> (212.319, -12.048)
  line L131 (104.919, -26.048) -> (118.919, -26.048)
  line L132 (62.879, -12.048) -> (48.879, -12.048)
  line L133 (216.999, -26.048) -> (230.999, -26.048)
  line L134 (230.999, -12.048) -> (216.999, -12.048)
  line L135 (76.899, -50.148) -> (75.461, -50.148)
  line L136 (123.599, -26.048) -> (137.599, -26.048)
  line L137 (156.279, -45.098) -> (156.279, -31.098)
  line L138 (174.959, -45.098) -> (174.959, -31.098)
  line L139 (160.959, -12.048) -> (160.959, -26.048)
  line L140 (-7.161, -45.098) -> (6.839, -45.098)
  line L141 (118.919, -31.098) -> (104.919, -31.098)
  line L142 (90.899, -64.148) -> (92.337, -64.148)
  line L143 (68.461, -64.148) -> (75.461, -64.148)
  line L144 (11.519, -31.098) -> (11.519, -45.098)
  line L145 (67.559, -31.098) -> (67.559, -45.098)
  line L146 (156.279, -12.048) -> (142.279, -12.048)
  line L147 (160.959, -26.048) -> (174.959, -26.048)
  line L148 (6.839, -64.148) -> (6.839, -50.148)
  line L149 (6.839, -50.148) -> (-7.161, -50.148)
  line L150 (174.959, -26.048) -> (174.959, -12.048)
  line L151 (100.239, -45.098) -> (100.239, -31.098)
  line L152 (174.959, -31.098) -> (160.959, -31.098)
  line L153 (25.519, -50.148) -> (11.519, -50.148)
  line L154 (212.319, -12.048) -> (198.319, -12.048)
  line L155 (216.999, -45.098) -> (230.999, -45.098)
  line L156 (123.599, -31.098) -> (123.599, -45.098)
  line L157 (51.269, -64.148) -> (52.009, -64.148)
  line L158 (156.279, -31.098) -> (142.279, -31.098)
  line L159 (142.279, -31.098) -> (142.279, -45.098)
  line L160 (179.639, -45.098) -> (193.639, -45.098)
  line L161 (30.199, -64.148) -> (44.199, -64.148)
  line L162 (75.461, -64.148) -> (76.899, -64.148)
  line L163 (198.319, -45.098) -> (212.319, -45.098)
  line L164 (142.279, -45.098) -> (156.279, -45.098)
  line L165 (58.269, -49.148) -> (52.009, -49.148)
  line L166 (44.199, -50.148) -> (30.199, -50.148)
  line L167 (92.337, -49.148) -> (90.109, -49.148)
  line L168 (59.009, -49.148) -> (58.269, -49.148)
  line L169 (92.337, -64.148) -> (97.109, -64.148)
  line L170 (90.109, -49.148) -> (90.109, -50.148)
  line L171 (97.109, -49.148) -> (92.337, -49.148)
  line L172 (212.319, -31.098) -> (198.319, -31.098)
  line L173 (230.999, 7.002) -> (216.999, 7.002)
  line L174 (6.839, 7.002) -> (-7.161, 7.002)
  line L175 (86.239, 7.002) -> (86.239, -6.998)
  line L176 (44.199, -6.998) -> (44.199, 7.002)
  line L177 (62.879, 7.002) -> (48.879, 7.002)
  line L178 (30.199, -6.998) -> (44.199, -6.998)
  line L179 (30.199, 7.002) -> (30.199, -6.998)
  line L180 (6.839, -6.998) -> (6.839, 7.002)
  line L181 (25.519, -6.998) -> (25.519, 7.002)
  line L182 (156.279, 7.002) -> (142.279, 7.002)
  line L183 (67.559, 7.002) -> (67.559, -6.998)
  line L184 (156.279, -6.998) -> (156.279, 7.002)
  line L185 (160.959, 7.002) -> (160.959, -6.998)
  line L186 (212.319, -6.998) -> (212.319, 7.002)
  line L187 (230.999, -6.998) -> (230.999, 7.002)
  line L188 (86.239, -6.998) -> (100.239, -6.998)
  line L189 (198.319, 7.002) -> (198.319, -6.998)
  line L190 (216.999, -6.998) -> (230.999, -6.998)
  line L191 (6.839, -12.048) -> (-7.161, -12.048)
  line L192 (216.999, 7.002) -> (216.999, -6.998)
  line L193 (25.519, -26.048) -> (25.519, -12.048)
  line L194 (30.199, -26.048) -> (44.199, -26.048)
  line L195 (142.279, -6.998) -> (156.279, -6.998)
  line L196 (104.919, 7.002) -> (104.919, -6.998)
  line L197 (11.519, -6.998) -> (25.519, -6.998)
  line L198 (160.959, -6.998) -> (174.959, -6.998)
  line L199 (142.279, 7.002) -> (142.279, -6.998)
  line L200 (11.519, -26.048) -> (25.519, -26.048)
  line L201 (179.639, 7.002) -> (179.639, -6.998)
  line L202 (6.839, -26.048) -> (6.839, -12.048)
  line L203 (11.519, -12.048) -> (11.519, -26.048)
  line L204 (193.639, 7.002) -> (179.639, 7.002)
  line L205 (48.879, -6.998) -> (62.879, -6.998)
  line L206 (25.519, -12.048) -> (11.519, -12.048)
  line L207 (100.239, 7.002) -> (86.239, 7.002)
  line L208 (-7.161, -12.048) -> (-7.161, -26.048)
  line L209 (-7.161, 7.002) -> (-7.161, -6.998)
  line L210 (104.919, -6.998) -> (118.919, -6.998)
  line L211 (174.959, 7.002) -> (160.959, 7.002)
  line L212 (193.639, -6.998) -> (193.639, 7.002)
  line L213 (-7.161, -6.998) -> (6.839, -6.998)
  line L214 (118.919, 7.002) -> (104.919, 7.002)
  line L215 (137.599, -6.998) -> (137.599, 7.002)
  line L216 (174.959, -6.998) -> (174.959, 7.002)
  line L217 (198.319, -6.998) -> (212.319, -6.998)
  line L218 (11.519, 7.002) -> (11.519, -6.998)
  line L219 (62.879, -6.998) -> (62.879, 7.002)
  line L220 (-7.161, -26.048) -> (6.839, -26.048)
  line L221 (81.559, 7.002) -> (67.559, 7.002)
  line L222 (25.519, 7.002) -> (11.519, 7.002)
  line L223 (118.919, -6.998) -> (118.919, 7.002)
  line L224 (48.879, 7.002) -> (48.879, -6.998)
  line L225 (123.599, 7.002) -> (123.599, -6.998)
  line L226 (137.599, 7.002) -> (123.599, 7.002)
  line L227 (123.599, -6.998) -> (137.599, -6.998)
  line L228 (212.319, 7.002) -> (198.319, 7.002)
  line L229 (44.199, 7.002) -> (30.199, 7.002)
  line L230 (100.239, -6.998) -> (100.239, 7.002)
  line L231 (81.559, -6.998) -> (81.559, 7.002)
  line L232 (179.639, -26.048) -> (193.639, -26.048)
  line L233 (81.559, -12.048) -> (67.559, -12.048)
  line L234 (137.599, -26.048) -> (137.599, -12.048)
  line L235 (6.839, -31.098) -> (-7.161, -31.098)
  line L236 (11.519, -45.098) -> (25.519, -45.098)
  line L237 (81.559, -26.048) -> (81.559, -12.048)
  line L238 (-7.161, -31.098) -> (-7.161, -45.098)
  line L239 (44.199, -12.048) -> (30.199, -12.048)
  line L240 (118.919, -26.048) -> (118.919, -12.048)
  line L241 (48.879, -12.048) -> (48.879, -26.048)
  line L242 (86.239, -26.048) -> (100.239, -26.048)
  line L243 (48.879, -26.048) -> (62.879, -26.048)
  line L244 (198.319, -12.048) -> (198.319, -26.048)
  line L245 (30.199, -45.098) -> (44.199, -45.098)
  line L246 (30.199, -12.048) -> (30.199, -26.048)
  line L247 (179.639, -6.998) -> (193.639, -6.998)
  line L248 (193.639, -12.048) -> (179.639, -12.048)
  line L249 (104.919, -12.048) -> (104.919, -26.048)
  line L250 (67.559, -6.998) -> (81.559, -6.998)
  line L251 (230.999, -26.048) -> (230.999, -12.048)
  line L252 (62.879, -31.098) -> (48.879, -31.098)
  line L253 (198.319, -26.048) -> (212.319, -26.048)
  line L254 (6.839, -45.098) -> (6.839, -31.098)
  line L255 (44.199, -31.098) -> (30.199, -31.098)
  line L256 (44.199, -26.048) -> (44.199, -12.048)
  line L257 (193.639, -26.048) -> (193.639, -12.048)
  line L258 (25.519, -31.098) -> (11.519, -31.098)
  line L259 (25.519, -45.098) -> (25.519, -31.098)
  line L260 (44.199, -45.098) -> (44.199, -31.098)
  line L261 (48.879, -45.098) -> (62.879, -45.098)
  line L262 (48.879, -31.098) -> (48.879, -45.098)
  line L263 (81.559, -45.098) -> (81.559, -31.098)
  line L264 (81.559, -31.098) -> (67.559, -31.098)
  line L265 (67.559, -45.098) -> (81.559, -45.098)